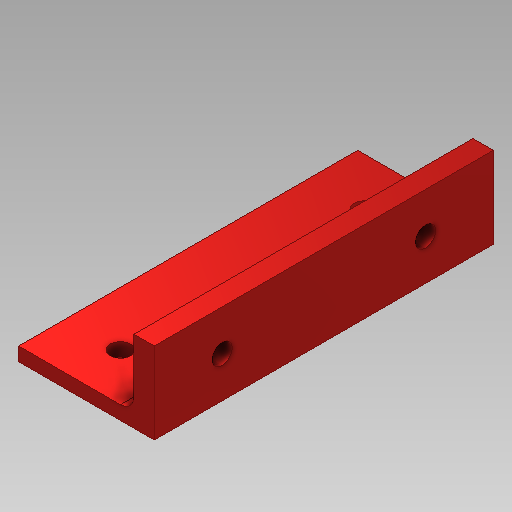
# Autodesk Inventor part: Sharp_IR_holder
Saved by Autodesk Inventor 2020 (Build 240168000, 168)
## iProperties
Created: 2022-08-18
Part Number: Sharp_IR_holder
Material: Aluminum, Anodized Red
Document SubType Name: Modeling
Designer: Umair
Density: 2.7 g/cm^3
Appearance: Anodized - Red
Author: Umair
Autodesk Inventor part; units mm, degrees
ref_plane "YZ Plane" through (0, 0, 0) normal (1, 0, 0) x (0, 1, 0)
ref_plane "XZ Plane" through (0, 0, 0) normal (0, 1, 0) x (-1, 0, 0)
ref_plane "XY Plane" through (0, 0, 0) normal (0, 0, 1) x (1, 0, 0)
sketch "Sketch1" plane through (0, 0, 0) normal (0, 1, 0) x (-1, 0, 0)
  line L0 (10, 25) -> (-10, 25)
  line L1 (-10, 25) -> (-10, -25)
  line L2 (-10, -25) -> (10, -25)
  line L3 (10, -25) -> (10, 25)
  line L4 (10, 25) -> (-10, -25) construction
  line L5 (-10, 25) -> (10, -25) construction
  line L6 (0, 0) -> (0, -18)
  line L7 (0, -18) -> (0, 18)
  line L8 (0, 18) -> (2, 18)
  line L9 (0, -18) -> (2, -18)
  circle A0 centre (2, 18) radius 1.5
  circle A1 centre (2, -18) radius 1.5
  dimension "d0" = 20
  dimension "d1" = 50
  dimension "d2" = 18
  dimension "d3" = 36
  dimension "d4" = 2
  dimension "d5" = 2
  dimension "d6" = 3
  dimension "d7" = 3
  constraints: 20 end point, 2 centre point, 2 coincident, 2 horizontal, 2 midpoint, 2 parallel, 2 perpendicular, 1 point on line, 1 vertical
  measures "d0" distance of L2.end L1.end
  measures "d1" distance of L1.end L0.end
  measures "d2" distance of L6.start L6.end
  measures "d3" distance of L6.end L7.end
  measures "d4" distance of L7.end L8.end
  measures "d5" distance of L6.end L9.end
  measures "d6" diameter of A0
  measures "d7" diameter of A1
extrude "Extrusion1" add sketch "Sketch1" against normal blind 2
sketch "Sketch2" plane through (0, 0, 0) normal (0, 1, 0) x (1, 0, 0)
  line L0 (10, 25) -> (10, -25) projected
  line L1 (10, -25) -> (7, -25)
  line L2 (10, -25) -> (-10, -25) projected
  line L3 (7, -25) -> (7, 25)
  line L4 (-10, 25) -> (10, 25) projected
  line L5 (7, 25) -> (10, 25)
  line L6 (10, 25) -> (10, -25)
  point P0 (0, 0)
  dimension "d10" = 3
  constraints: 8 end point, 2 collinear, 1 point on line, 1 vertical
  measures "d10" distance of L0.end L1.end
extrude "Extrusion2" add sketch "Sketch2" along normal blind 10
sketch "Sketch3" plane through (10, -2, 25) normal (1, 0, 0) x (0, 0, -1)
  line L0 (50, 0) -> (0, 0) projected
  line L1 (25, 0) -> (25, 6)
  line L2 (25, 6) -> (45, 6)
  line L3 (45, 6) -> (25, 6)
  line L4 (25, 6) -> (5, 6)
  line L5 (5, 6) -> (10, 6)
  line L6 (10, 6) -> (40, 6)
  circle A0 centre (40, 6) radius 1.5
  circle A1 centre (10, 6) radius 1.5
  point P0 (25, 2)
  dimension "d13" = 6
  dimension "d14" = 20
  dimension "d15" = 20
  dimension "d16" = 20
  dimension "d17" = 5
  dimension "d18" = 30
  dimension "d19" = 3
  dimension "d20" = 3
  constraints: 12 end point, 3 point on line, 2 centre point, 2 coincident, 1 collinear, 1 midpoint, 1 perpendicular, 1 vertical
  measures "d13" distance of L1.start L1.end
  measures "d14" distance of L1.end L2.end
  measures "d15" distance of L2.end L1.end
  measures "d16" distance of L1.end L4.end
  measures "d17" distance of L4.end L5.end
  measures "d18" distance of L5.end L6.end
  measures "d19" diameter of A0
  measures "d20" diameter of A1
extrude "Extrusion3" cut sketch "Sketch3" against normal blind 10
fillet "Fillet1" radius 2 1 edges at (7, 0, 0)
body "Solid1"
